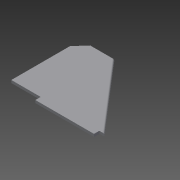
# Autodesk Inventor part: vertikal stab
Saved by Autodesk Inventor 2014 SP1 (Build 180222100, 222)
## iProperties
Created: 2018-05-07
Part Number: vertikal stab
Material: Generic
Document SubType Name: Modeling
Designer: Dadang
Density: 1 g/cm^3
Appearance: Default
Author: Dadang
Autodesk Inventor part; units mm, degrees
ref_plane "YZ Plane" through (0, 0, 0) normal (1, 0, 0) x (0, 1, 0)
ref_plane "XZ Plane" through (0, 0, 0) normal (0, 1, 0) x (-1, 0, 0)
ref_plane "XY Plane" through (0, 0, 0) normal (0, 0, 1) x (1, 0, 0)
sketch "Sketch1" plane through (0, 0, 0) normal (0, 0, 1) x (1, 0, 0)
  line L0 (0, 0) -> (0, 110)
  line L1 (18, 130) -> (0, 110)
  line L2 (18, 130) -> (63, 130)
  line L3 (0, 0) -> (175, 0)
  line L4 (175, 0) -> (63, 130)
  line L5 (165, 0) -> (165, -10)
  line L6 (165, -10) -> (55, -10)
  line L7 (55, -10) -> (55, 0)
  dimension "d1" = 110
  dimension "d5" = 45
  dimension "d6" = 175
  dimension "d7" = 10
  dimension "d8" = 10
  dimension "d9" = 110
  constraints: 16 end point, 3 perpendicular, 2 parallel, 2 point on line
  measures "d1" distance of L0.start L0.end
  measures "d5" distance of L1.start L2.end
  measures "d6" distance of L0.start L3.end
  measures "d7" distance of L3.end L5.start
  measures "d8" distance of L5.start L5.end
  measures "d9" distance of L5.end L6.end
extrude "Extrusion1" add sketch "Sketch1" along normal blind 5
fillet "Fillet1" radius 2.5 2 edges at (119, 65, 5) (119, 65, 0)
body "Solid1"
